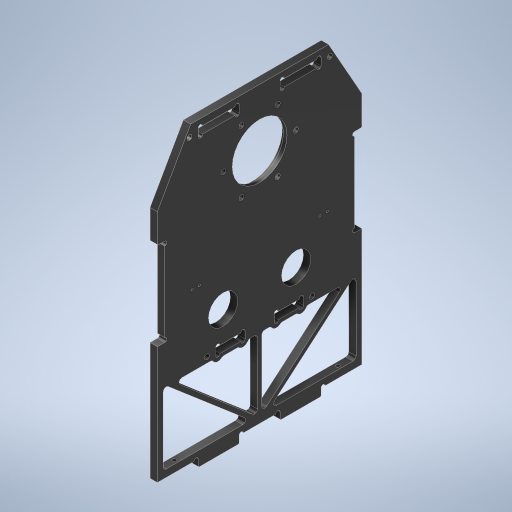
# Autodesk Inventor part: TorsoSideFrame_
Saved by Autodesk Inventor 2024.2 (Build 282272000, 272)
## iProperties
Created: 2024-01-27
Part Number: TorsoSideFrame_
Material: Aluminum 7075
Document SubType Name: Modeling
Designer: Masato Kubotera
Density: 2.81 g/cm^3
Appearance: Glossy - Black
Mass: 218.963 g
Surface Area: 501.509 cm^2
Volume: 77.9229 cm^3
Vendor: meviy
Author: Masato Kubotera
Autodesk Inventor part; units mm, degrees
ref_plane "YZ Plane" through (0, 0, 0) normal (1, 0, 0) x (0, 1, 0)
ref_plane "XZ Plane" through (0, 0, 0) normal (0, 1, 0) x (-1, 0, 0)
ref_plane "XY Plane" through (0, 0, 0) normal (0, 0, 1) x (1, 0, 0)
sketch "Sketch1" plane through (0, 0, 0) normal (0, 1, 0) x (-1, 0, 0)
  circle A0 centre (0, 0) radius 18.75
  line L0 (0, 0) -> (0, -161.5)
  circle A1 centre (0, 0) radius 29 construction
  line L1 (0, 0) -> (0, 39.5)
  line L2 (0, 39.5) -> (-47.1831, 39.5)
  line L3 (-70, -1) -> (-70, -106.5)
  line L4 (-70, -161.5) -> (-42, -161.5)
  line L5 (-42, -161.5) -> (-42, -166.5)
  line L6 (-42, -166.5) -> (-14, -166.5)
  line L7 (-14, -166.5) -> (-14, -161.5)
  line L8 (-14, -161.5) -> (0, -161.5)
  line L9 (-65, -20.95) -> (-70, -20.95)
  line L10 (-56, -161.5) -> (-56, -155.5) construction
  line L11 (-28, -166.5) -> (-28, -161.5) construction
  arc A2 (-11, -161.5) -> (-14, -161.5) centre (-12.5, -161.5) ccw
  arc A3 (-42, -161.5) -> (-45, -161.5) centre (-43.5, -161.5) ccw
  line L12 (-70, -1) -> (-65, -1) construction
  line L13 (-65, -1) -> (-65, -106.5) construction
  line L14 (-67.5, -1) -> (-67.5, -106.5) construction
  line L15 (-70, -66) -> (0, -66) construction
  line L16 (-70, -21) -> (-65, -21) construction
  arc A4 (-65, -23.95) -> (-65, -20.95) centre (-65, -22.45) ccw
  line L17 (-65, -106.5) -> (0, -106.5) construction
  line L18 (-65, -101.5) -> (0, -101.5) construction
  line L19 (-65, -104) -> (-20, -104) construction
  line L20 (-9.95, -106.55) -> (-30.05, -106.55)
  line L21 (-30.05, -106.55) -> (-30.05, -101.45)
  line L22 (-30.05, -101.45) -> (-9.95, -101.45)
  line L23 (-9.95, -101.45) -> (-9.95, -106.55)
  line L24 (-9.95, -106.55) -> (-30.05, -101.45) construction
  line L25 (-30.05, -106.55) -> (-9.95, -101.45) construction
  line L26 (-30, -101.5) -> (-30, -106.5) construction
  arc A5 (-27.05, -101.45) -> (-30.05, -101.45) centre (-28.55, -101.45) ccw
  arc A6 (-30.05, -106.55) -> (-27.05, -106.55) centre (-28.55, -106.55) ccw
  line L27 (-15, -71.5) -> (-35, -71.5) construction
  line L28 (-35, -71.5) -> (-35, -91.5) construction
  line L29 (-35, -91.5) -> (-15, -91.5) construction
  line L30 (-15, -91.5) -> (-15, -71.5) construction
  line L31 (-15, -71.5) -> (-35, -91.5) construction
  line L32 (-35, -71.5) -> (-15, -91.5) construction
  line L33 (-37.5, -69) -> (-12.5, -69) construction
  line L34 (-12.5, -69) -> (-12.5, -94) construction
  line L35 (-12.5, -94) -> (-37.5, -94) construction
  line L36 (-37.5, -94) -> (-37.5, -69) construction
  line L37 (-37.5, -69) -> (-12.5, -94) construction
  line L38 (-12.5, -69) -> (-37.5, -94) construction
  line L39 (-50, 34.5) -> (0, 34.5) construction
  line L40 (-42.05, 34.55) -> (-13.95, 34.55)
  line L41 (-13.95, 34.55) -> (-13.95, 29.45)
  line L42 (-13.95, 29.45) -> (-42.05, 29.45)
  line L43 (-42.05, 29.45) -> (-42.05, 34.55)
  line L44 (-42.05, 34.55) -> (-13.95, 29.45) construction
  line L45 (-13.95, 34.55) -> (-42.05, 29.45) construction
  line L46 (-42.05, 32) -> (-13.95, 32) construction
  line L47 (-42, 34.5) -> (-42, 29.5) construction
  line L48 (-28, 34.55) -> (-28, 29.45) construction
  line L49 (-14, 34.5) -> (-14, 29.5) construction
  arc A7 (-39.05, 34.55) -> (-42.05, 34.55) centre (-40.55, 34.55) ccw
  arc A8 (-42.05, 29.45) -> (-39.05, 29.45) centre (-40.55, 29.45) ccw
  arc A9 (-13.95, 34.55) -> (-16.95, 34.55) centre (-15.45, 34.55) ccw
  arc A10 (-16.95, 29.45) -> (-13.95, 29.45) centre (-15.45, 29.45) ccw
  line L50 (-54.4689, -111.271) -> (-4.7987, -153.6833)
  line L51 (-65.9501, -109.75) -> (-65.9501, -154.5)
  line L52 (-63.9501, -156.5) -> (-11.5422, -156.5)
  line L53 (-10.2434, -152.979) -> (-62.6514, -108.229)
  arc A11 (-62.6514, -108.229) -> (-65.9501, -109.75) centre (-63.9501, -109.75) ccw
  arc A12 (-65.9501, -154.5) -> (-63.9501, -156.5) centre (-63.9501, -154.5) ccw
  arc A13 (-11.5422, -156.5) -> (-10.2434, -152.979) centre (-11.5422, -154.5) ccw
  line L54 (-61.4895, -100.25) -> (-33.6254, -100.25)
  circle A14 centre (-46.25, -59) radius 3 construction
  line L55 (-1.5, -56) -> (-61.4895, -56)
  line L56 (0, 0) -> (-29, 0) construction
  line L57 (-40.95, 23.9454) -> (-40.95, -23.9454)
  line L58 (-53.1702, -107.75) -> (-33.6254, -107.75)
  arc A15 (-31.9336, -108.6833) -> (-25.8669, -109.5167) centre (-28.55, -106.55) ccw
  line L59 (-1.5, -152.1623) -> (-1.5, -109.75)
  arc A16 (-53.1702, -107.75) -> (-54.4689, -111.271) centre (-53.1702, -109.75) ccw
  arc A17 (-1.5, -109.75) -> (-3.5, -107.75) centre (-3.5, -109.75) ccw
  arc A18 (-31.9336, -108.6833) -> (-33.6254, -107.75) centre (-33.6254, -109.75) ccw
  circle A19 centre (-36, -104) radius 1.75 construction
  arc A20 (-24.5254, -109) -> (-25.8669, -109.5167) centre (-24.5254, -111) ccw
  line L60 (-47.1831, 39.5) -> (-70, -1)
  line L61 (-46.582, -26.0941) -> (-61.4895, -26.0941)
  line L62 (-20, -101.45) -> (-20, -106.55) construction
  arc A21 (-25.8669, -98.4833) -> (-31.9336, -99.3167) centre (-28.55, -101.45) ccw
  arc A22 (-33.6254, -100.25) -> (-31.9336, -99.3167) centre (-33.6254, -98.25) ccw
  arc A23 (-25.8669, -98.4833) -> (-24.5254, -99) centre (-24.5254, -97) ccw
  line L63 (-10, -101.5) -> (-10, -106.5) construction
  arc A24 (-9.95, -101.45) -> (-12.95, -101.45) centre (-11.45, -101.45) ccw
  arc A25 (-12.95, -106.55) -> (-9.95, -106.55) centre (-11.45, -106.55) ccw
  arc A26 (-14.1331, -109.5167) -> (-8.0664, -108.6833) centre (-11.45, -106.55) ccw
  arc A27 (-6.3746, -107.75) -> (-8.0664, -108.6833) centre (-6.3746, -109.75) ccw
  arc A28 (-14.1331, -109.5167) -> (-15.4746, -109) centre (-15.4746, -111) ccw
  arc A29 (-8.0664, -99.3167) -> (-6.3746, -100.25) centre (-6.3746, -98.25) ccw
  arc A30 (-8.0664, -99.3167) -> (-14.1331, -98.4833) centre (-11.45, -101.45) ccw
  arc A31 (-15.4746, -99) -> (-14.1331, -98.4833) centre (-15.4746, -97) ccw
  line L64 (-24.5254, -99) -> (-15.4746, -99)
  line L65 (-24.5254, -109) -> (-15.4746, -109)
  line L66 (-6.3746, -107.75) -> (-3.5, -107.75)
  arc A32 (-3.5, -100.25) -> (-1.5, -98.25) centre (-3.5, -98.25) ccw
  line L67 (-6.3746, -100.25) -> (-3.5, -100.25)
  line L68 (-46.25, -59) -> (-41.25, -59) construction
  line L69 (-65, -23.95) -> (-65, -78.05)
  line L70 (-65, -51) -> (-70, -51) construction
  line L71 (-65, -81.05) -> (-70, -81.05)
  line L72 (-70, -81) -> (-65, -81) construction
  arc A33 (-65, -81.05) -> (-65, -78.05) centre (-65, -79.55) ccw
  line L73 (-65, -106.5) -> (-70, -106.5) construction
  line L74 (-1.5, -22.4499) -> (-1.5, -56)
  line L75 (-61.4895, -62) -> (-1.5, -62)
  line L76 (-1.5, -62) -> (-1.5, -98.25)
  line L77 (-61.4895, -56) -> (-61.4895, -26.0941)
  circle A34 centre (-25, -81.5) radius 10
  line L78 (-61.4895, -62) -> (-61.4895, -100.25)
  arc A35 (-4.7987, -153.6833) -> (-1.5, -152.1623) centre (-3.5, -152.1623) ccw
  circle A36 centre (-25, -81.5) radius 11
  arc A37 (-14.0872, 17.5443) -> (-22.2374, 3.4277) centre (0, 0) ccw
  arc A38 (-22.2374, -3.4277) -> (-14.0872, -17.5443) centre (0, 0) ccw
  arc A39 (-8.1502, -20.972) -> (-1.5, -22.4499) centre (0, 0) ccw
  arc A40 (-14.0872, -17.5443) -> (-8.1502, -20.972) centre (-12.375, -21.4341) ccw
  arc A41 (-22.2374, 3.4277) -> (-22.2374, -3.4277) centre (-24.75, 0) ccw
  arc A42 (-10.9839, 25.45) -> (-14.0872, 17.5443) centre (-12.375, 21.4341) ccw
  line L79 (-70, -106.5) -> (-70, -161.5)
  point P0 (-16.05, -9.6933)
  point P1 (12.375, -21.4341)
  point P2 (24.75, 0)
  point P3 (12.375, 21.4341)
  point P4 (-28, 32)
  point P5 (0, -130.75)
  point P6 (-45.6341, -118.8149)
  point P7 (0, -157.7808)
  point P8 (0, -18.75)
  point P9 (0, 18.75)
  point P10 (0, -106.55)
  point P11 (-27.05, -106.55)
  point P12 (0, -101.45)
  point P13 (-16.95, 29.45)
  point P14 (-39.05, 29.45)
  point P15 (-16.95, 34.55)
  point P16 (-48, 32)
  point P17 (-35.05, 18.95)
  point P18 (-53.9811, -94)
  point P19 (-1.5, -156.5)
  point P20 (-7, -161.5)
  point P21 (-66.3533, -107.75)
  point P22 (-32.3658, -107.75)
  point P23 (-32.5089, -107.1221)
  point P24 (-7.6342, -107.75)
  point P25 (-12.95, -101.45)
  point P26 (-12.95, -106.55)
  point P27 (-42, 32)
  dimension "d0" = 37.5
  dimension "d1" = 161.5
  dimension "d2" = 58
  dimension "d16" = 360
  dimension "d18" = 49.5
  dimension "d19" = 140
  dimension "d20" = 28
  dimension "d21" = 5
  dimension "d22" = 28
  dimension "d23" = 6
  dimension "d24" = 0.05
  dimension "d26" = 5
  dimension "d27" = 21.25
  dimension "d30" = 55
  dimension "d31" = 5
  dimension "d32" = 55
  dimension "d34" = 0.05
  dimension "d35" = 1.5
  dimension "d36" = 0.05
  dimension "d37" = 6
  dimension "d38" = 20
  dimension "d39" = 20
  dimension "d40" = 25
  dimension "d41" = 25
  dimension "d52" = 0.05
  dimension "d53" = 0.05
  dimension "d54" = 2
  dimension "d58" = 3
  dimension "d105" = 6
  dimension "d108" = 6
  dimension "d130" = 5
  dimension "d134" = 2
  dimension "d136" = 3.5
  dimension "d137" = 2
  dimension "d142" = 3
  dimension "d156" = 2.5
  dimension "d157" = 2.5
  dimension "d158" = 20
  dimension "d160" = 60
  dimension "d162" = 5
  dimension "d163" = 105.5
  dimension "d164" = 50
  dimension "d165" = 40.5
  dimension "d166" = 50
  dimension "d167" = 20
  dimension "d169" = 50
  dimension "d170" = 20
  dimension "d171" = 20
  dimension "d172" = 45
  dimension "d180" = 1
  dimension "d181" = 22.5
  dimension "d182" = 5
  dimension "d183" = 10
  dimension "d184" = 201
  constraints: 161 end point, 78 point on circle, 45 symmetric about line, 42 centre point, 41 point on line, 25 horizontal, 24 tangent, 22 midpoint, 18 vertical, 14 coincident, 10 equal radius, 10 parallel, 7 collinear, 4 perpendicular, 30 other
  measures "d1" distance of L0.start L0.end
  measures "d2" diameter of A1
  measures "d18" distance of point (24.75, 0) point (-24.75, 0)
  measures "d19" diameter of L4.start L0
  measures "d20" diameter of L7 L0
  measures "d21" distance of L4.end L5.end
  measures "d22" distance from line of L5 L4.start
  measures "d23" distance of L10.start L10.end
  measures "d24" distance between parallel lines of L9 L16
  measures "d26" distance of point (-41.25, -59) point (-46.25, -59)
  measures "d27" distance from line of point (-46.25, -59) L14
  measures "d30" distance from line of L3.end L4
  measures "d31" distance between parallel lines of L17 L18
  measures "d32" distance between parallel lines of L4 L17
  measures "d34" distance between parallel lines of L18 L22
  measures "d35" radius of A4
  measures "d36" distance between parallel lines of L21 L26
  measures "d37" distance from line of L26 point (-36, -104)
  measures "d38" distance of L29.end L28.end
  measures "d39" distance of L28.end L27.end
  measures "d40" distance of L34.end L35.end
  measures "d41" distance of L33.end L34.end
  measures "d52" distance between parallel lines of L43 L47
  measures "d53" distance between parallel lines of L40 L39
  measures "d54" radius of A11
  measures "d58" distance between parallel lines of L53 L50
  measures "d105" diameter of A14
  measures "d108" distance from line of point (-48, 32) L47
  measures "d130" distance from line of point (-7, -161.5) L52
  measures "d134" radius of A16
  measures "d136" diameter of A19
  measures "d137" distance edge to line of A19 L58
  measures "d142" diameter of L59 L0
  measures "d156" distance between parallel lines of L65 L17
  measures "d157" radial gap between concentric circles of A15 A6
  measures "d158" distance between parallel lines of L63 L26
  measures "d160" distance between parallel lines of L72 L16
  measures "d162" distance of L13.end L73.end
  measures "d163" distance of L3.start L73.end
  measures "d164" distance of L70.end L3.start
  measures "d165" vertical distance of L3.start L2.end
  measures "d166" distance of L39.start L39.end
  measures "d167" diameter of L63 L0
  measures "d169" diameter of point (-25, -81.5) L0
  measures "d170" distance from line of L18 point (-25, -81.5)
  measures "d171" diameter of A34
  measures "d172" distance between parallel lines of L19 L68
  measures "d180" radial gap between concentric circles of A36 A34
  measures "d181" radius of A37
  measures "d182" distance of L47.start L47.end
  measures "d183" distance from line of L47.end L2
  measures "d184" distance between parallel lines of L2 L4
extrude "Extrusion1" add sketch "Sketch1" along normal blind 5 contours A0 L0 L8 A2 L7 L6 L5 A3 L4 L79 L3 L71 A33 L69 A4 L9 L60 L2 L1 | L78 L75 L76 A32 L67 A29 A30 A31 L64 A23 A21 A22 L54 | A36
extrude "Extrusion3" cut sketch "Sketch1" along normal blind 4 contours L78 L75 L76 A32 L67 A29 A30 A31 L64 A23 A21 A22 L54
hole "Hole1" at (24.75, 0, 0) at (12.375, 0, -21.4341) at (-12.375, 0, -21.4341) at (12.375, 0, 21.4341) direction (0, 1, 0) diameter 3.5 end through all counterbore diameter 6.1 counterbore depth 3.5
hole "Hole2" at (46.25, 0, -59) at (41.25, 0, -59) direction (0, 1, 0) diameter 1.567 end through all thread size "M2x0.4" class "6H" standard "ANSI Metric M Profile"
hole "Hole3" at (36, 0, -104) at (48, 0, 32) direction (0, 1, 0) diameter 3.5 end through all
sketch "Sketch2" plane through (70, 0, -161.5) normal (0, 0, -1) x (-1, 0, 0)
  line L0 (0, 5) -> (28, 5) projected
  line L1 (14, 5) -> (14, 0)
  line L2 (0, 0) -> (28, 0) projected
  line L3 (70, 0) -> (70, 5) projected
  point P0 (14, 2.5)
  point P1 (70, 2.5)
  constraints: 3 midpoint, 2 end point, 1 perpendicular, 1 vertical
hole "Hole5" at (56, 2.5, -161.5) at (0, 2.5, -161.5) direction (0, 0, 1) diameter 2.459 depth 6 thread size "M3x0.5" class "6H" standard "ANSI Metric M Profile"
hole "Hole6" at (0, 0, 0) direction (0, 1, 0) diameter 41 depth 2.5
chamfer "Chamfer1" distance 0.5 angle 45 3 edges at (70, 2.5, -20.95) (42, 2.5, -166.5) (14, 2.5, -166.5)
fillet "Fillet1" radius 2.5 3 edges at (61.4895, 2, -100.25) (1.5, 2, -62) (61.4895, 2, -62)
fillet "Fillet2" [suppressed]
mirror "Mirror1" about plane through (0, 0, 0) normal (1, 0, 0)
body "Solid1"
